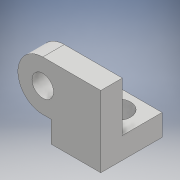
# Autodesk Inventor part: P3-12
Saved by Autodesk Inventor 2017 (Build 210142000, 142)
## iProperties
Created: 2017-02-12
Part Number: P3-12
Material: Generic
Document SubType Name: Modeling
Designer: Schaffel
Density: 1 g/cm^3
Appearance: Default
Author: Schaffel
Autodesk Inventor part; units mm, degrees
ref_plane "YZ Plane" through (0, 0, 0) normal (1, 0, 0) x (0, 1, 0)
ref_plane "XZ Plane" through (0, 0, 0) normal (0, 1, 0) x (-1, 0, 0)
ref_plane "XY Plane" through (0, 0, 0) normal (0, 0, 1) x (1, 0, 0)
sketch "Sketch1" plane through (0, 0, 0) normal (0, 0, 1) x (1, 0, 0)
  line L0 (0, 0) -> (50, 0)
  line L1 (50, 0) -> (50, 13)
  line L2 (50, 13) -> (0, 13)
  line L3 (0, 13) -> (0, 0)
  dimension "d0" = 50
  constraints: 8 end point, 3 perpendicular, 1 horizontal
  measures "d0" distance of L0.start L0.end
extrude "Extrusion1" add sketch "Sketch1" along normal blind 30
fillet "Fillet1" radius 15 2 edges at (0, 6.5, 30) (0, 6.5, 0)
sketch "Sketch2" plane through (50, 0, 0) normal (0, -1, 0) x (1, 0, 0)
  line L0 (0, 0) -> (-35, 0) projected
  line L1 (0, 0) -> (-30, 0)
  line L2 (-30, 0) -> (-30, -13)
  line L3 (-30, -13) -> (0, -13)
  line L4 (0, -13) -> (0, 0)
  point P0 (-50, 0)
  constraints: 8 end point, 2 perpendicular, 1 point on line, 1 vertical
extrude "Extrusion2" add sketch "Sketch2" against normal blind 37
sketch "Sketch3" plane through (15, 13, 30) normal (0, 1, 0) x (1, 0, 0)
  arc A0 (0, 30) -> (0, 0) centre (0, 15) ccw projected
  circle A1 centre (0, 15) radius 6.5
  point P0 (-15, 30)
  dimension "d6" = 13
  constraints: 1 centre point, 1 coincident
  measures "d6" diameter of A1
extrude "Extrusion3" cut sketch "Sketch3" against normal blind 37
sketch "Sketch4" plane through (20, 13, 0) normal (0, 0, 1) x (1, 0, 0)
  circle A0 centre (15, 12) radius 8
  point P0 (-20, -13)
  constraints: 1 centre point
extrude "Extrusion4" cut sketch "Sketch4" against normal blind 13
body "Solid1"
